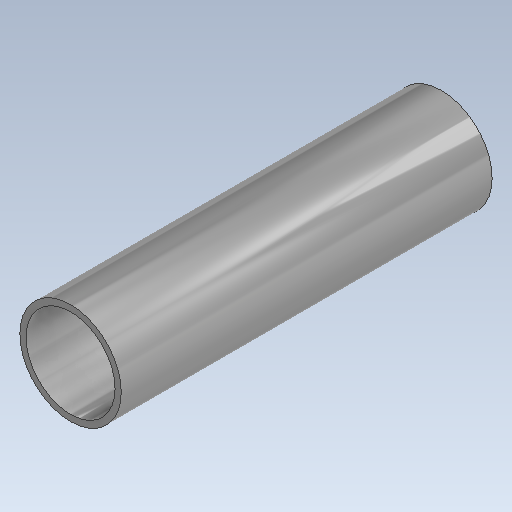
# Autodesk Inventor part: ZALC18210
Saved by Autodesk Inventor 2021 (Build 250183000, 183)
## iProperties
RuleStatus: InUse
Created: 2020-04-29
Part Number: ZALC18210
Material: Aluminium 7005 T6
Document SubType Name: Modeling
Designer: Hannah
Density: 2.7 g/cm^3
Appearance: Aluminum - Polished
Mass: 122.463 g
Surface Area: 368.902 cm^2
Volume: 45.3567 cm^3
Vendor: Ceeway
Catalog Web Link: https://www.framebuilding.com/ZONAL.htm
Description: head tube
OD: 41.0
Length: 150.0
Size: [7]
Author: Hannah
Revision Number: -
Autodesk Inventor part; units mm, degrees
ref_plane "YZ Plane" through (0, 0, 0) normal (1, 0, 0) x (0, 1, 0)
ref_plane "XZ Plane" through (0, 0, 0) normal (0, 1, 0) x (-1, 0, 0)
ref_plane "XY Plane" through (0, 0, 0) normal (0, 0, 1) x (1, 0, 0)
sketch "Sketch1" plane through (0, 0, 0) normal (0, 0, 1) x (1, 0, 0)
  circle A0 centre (0, 0) radius 18
  circle A1 centre (0, 0) radius 20.5
  dimension "d0" = 36
  dimension "OD" = 41
  constraints: 2 centre point, 2 coincident
  measures "d0" diameter of A0
  measures "OD" diameter of A1
extrude "Extrusion1" add sketch "Sketch1" along normal mid plane 150
body "Solid1"
